Autodesk Fusion 360 part; units mm, degrees
(part 2 of 2)
  arc A367 (268.1669, -101.5666) -> (267.6669, -101.0666) centre (267.6669, -101.5666) ccw
  arc A368 (269.9703, -102.354) -> (269.4703, -101.854) centre (269.4703, -102.354) ccw
  arc A369 (269.9703, -102.5224) -> (270.4703, -103.0224) centre (270.4703, -102.5224) ccw
  arc A370 (272.5183, -103.0224) -> (273.0183, -102.5224) centre (272.5183, -102.5224) ccw
  arc A371 (273.5183, -101.854) -> (273.0183, -102.354) centre (273.5183, -102.354) ccw
  arc A372 (274.3216, -101.854) -> (274.8216, -101.354) centre (274.3216, -101.354) ccw
  arc A373 (275.3216, -95.758) -> (274.8216, -96.258) centre (275.3216, -96.258) ccw
  arc A374 (275.6852, -93.464) -> (275.1852, -92.964) centre (275.1852, -93.464) ccw
  arc A375 (274.8216, -90.0604) -> (274.3216, -89.5604) centre (274.3216, -90.0604) ccw
  line L406 (293.5375, -88.25) -> (306.5375, -88.25)
  line L407 (293.5375, -102.25) -> (306.5375, -102.25)
  line L408 (293.0375, -88.75) -> (293.0375, -101.75)
  line L409 (307.0375, -88.75) -> (307.0375, -101.75)
  arc A376 (293.5375, -88.25) -> (293.0375, -88.75) centre (293.5375, -88.75) ccw
  arc A377 (307.0375, -88.75) -> (306.5375, -88.25) centre (306.5375, -88.75) ccw
  arc A378 (293.0375, -101.75) -> (293.5375, -102.25) centre (293.5375, -101.75) ccw
  arc A379 (306.5375, -102.25) -> (307.0375, -101.75) centre (306.5375, -101.75) ccw
  line L410 (312.5875, -88.25) -> (325.5875, -88.25)
  line L411 (312.5875, -102.25) -> (325.5875, -102.25)
  line L412 (312.0875, -88.75) -> (312.0875, -101.75)
  line L413 (326.0875, -88.75) -> (326.0875, -101.75)
  arc A380 (312.5875, -88.25) -> (312.0875, -88.75) centre (312.5875, -88.75) ccw
  arc A381 (326.0875, -88.75) -> (325.5875, -88.25) centre (325.5875, -88.75) ccw
  arc A382 (312.0875, -101.75) -> (312.5875, -102.25) centre (312.5875, -101.75) ccw
  arc A383 (325.5875, -102.25) -> (326.0875, -101.75) centre (325.5875, -101.75) ccw
  line L414 (331.6375, -88.25) -> (344.6375, -88.25)
  line L415 (331.6375, -102.25) -> (344.6375, -102.25)
  line L416 (331.1375, -88.75) -> (331.1375, -101.75)
  line L417 (345.1375, -88.75) -> (345.1375, -101.75)
  arc A384 (331.6375, -88.25) -> (331.1375, -88.75) centre (331.6375, -88.75) ccw
  arc A385 (345.1375, -88.75) -> (344.6375, -88.25) centre (344.6375, -88.75) ccw
  arc A386 (331.1375, -101.75) -> (331.6375, -102.25) centre (331.6375, -101.75) ccw
  arc A387 (344.6375, -102.25) -> (345.1375, -101.75) centre (344.6375, -101.75) ccw
  line L418 (5.4062, -107.3) -> (18.4063, -107.3)
  line L419 (5.4062, -121.3) -> (18.4063, -121.3)
  line L420 (4.9062, -107.8) -> (4.9062, -120.8)
  line L421 (18.9062, -107.8) -> (18.9062, -120.8)
  arc A388 (5.4062, -107.3) -> (4.9062, -107.8) centre (5.4062, -107.8) ccw
  arc A389 (18.9062, -107.8) -> (18.4062, -107.3) centre (18.4062, -107.8) ccw
  arc A390 (4.9062, -120.8) -> (5.4062, -121.3) centre (5.4062, -120.8) ccw
  arc A391 (18.4062, -121.3) -> (18.9063, -120.8) centre (18.4062, -120.8) ccw
  line L422 (29.2188, -107.3) -> (42.2188, -107.3)
  line L423 (29.2188, -121.3) -> (42.2188, -121.3)
  line L424 (28.7188, -107.8) -> (28.7188, -120.8)
  line L425 (42.7188, -107.8) -> (42.7188, -120.8)
  arc A392 (29.2188, -107.3) -> (28.7187, -107.8) centre (29.2188, -107.8) ccw
  arc A393 (42.7188, -107.8) -> (42.2188, -107.3) centre (42.2188, -107.8) ccw
  arc A394 (28.7188, -120.8) -> (29.2188, -121.3) centre (29.2188, -120.8) ccw
  arc A395 (42.2188, -121.3) -> (42.7188, -120.8) centre (42.2188, -120.8) ccw
  line L426 (53.0313, -107.3) -> (66.0312, -107.3)
  line L427 (53.0313, -121.3) -> (66.0312, -121.3)
  line L428 (52.5313, -107.8) -> (52.5313, -120.8)
  line L429 (66.5312, -107.8) -> (66.5312, -120.8)
  arc A396 (53.0313, -107.3) -> (52.5312, -107.8) centre (53.0313, -107.8) ccw
  arc A397 (66.5312, -107.8) -> (66.0312, -107.3) centre (66.0312, -107.8) ccw
  arc A398 (52.5313, -120.8) -> (53.0313, -121.3) centre (53.0313, -120.8) ccw
  arc A399 (66.0312, -121.3) -> (66.5312, -120.8) centre (66.0312, -120.8) ccw
  line L430 (124.4688, -107.3) -> (137.4688, -107.3)
  line L431 (124.4688, -121.3) -> (137.4688, -121.3)
  line L432 (123.9688, -107.8) -> (123.9688, -120.8)
  line L433 (137.9688, -107.8) -> (137.9688, -120.8)
  arc A400 (124.4688, -107.3) -> (123.9688, -107.8) centre (124.4688, -107.8) ccw
  arc A401 (137.9688, -107.8) -> (137.4688, -107.3) centre (137.4688, -107.8) ccw
  arc A402 (123.9688, -120.8) -> (124.4688, -121.3) centre (124.4688, -120.8) ccw
  arc A403 (137.4688, -121.3) -> (137.9688, -120.8) centre (137.4688, -120.8) ccw
  line L434 (78.1414, -108.6104) -> (83.7961, -108.6104)
  line L435 (84.2961, -109.1104) -> (84.2961, -111.5)
  line L436 (84.7962, -112) -> (130.9688, -112)
  line L437 (130.9688, -116.6) -> (84.7961, -116.6)
  line L438 (84.2961, -117.1) -> (84.2961, -120.404)
  line L439 (83.7961, -120.904) -> (82.9928, -120.904)
  line L440 (82.4928, -121.404) -> (82.4928, -121.5724)
  line L441 (81.9928, -122.0724) -> (79.9447, -122.0724)
  line L442 (79.4447, -121.5724) -> (79.4447, -121.404)
  line L443 (78.9447, -120.904) -> (78.1414, -120.904)
  line L444 (77.6414, -120.404) -> (77.6414, -115.308)
  line L445 (77.1414, -114.808) -> (76.7777, -114.808)
  line L446 (76.7777, -114.808) -> (76.7777, -112.514)
  line L447 (77.2777, -112.014) -> (77.6414, -112.014)
  line L448 (77.6414, -112.014) -> (77.6414, -109.1104)
  arc A404 (84.2962, -109.1104) -> (83.7961, -108.6104) centre (83.7961, -109.1104) ccw
  arc A405 (84.2962, -111.5) -> (84.7962, -112) centre (84.7962, -111.5) ccw
  arc A406 (84.7962, -116.6) -> (84.2962, -117.1) centre (84.7962, -117.1) ccw
  arc A407 (83.7961, -120.904) -> (84.2962, -120.404) centre (83.7961, -120.404) ccw
  arc A408 (82.9928, -120.904) -> (82.4928, -121.404) centre (82.9928, -121.404) ccw
  arc A409 (81.9928, -122.0724) -> (82.4927, -121.5724) centre (81.9928, -121.5724) ccw
  arc A410 (79.4447, -121.5724) -> (79.9447, -122.0724) centre (79.9447, -121.5724) ccw
  arc A411 (79.4447, -121.404) -> (78.9447, -120.904) centre (78.9447, -121.404) ccw
  arc A412 (77.6414, -120.404) -> (78.1414, -120.904) centre (78.1414, -120.404) ccw
  arc A413 (77.6414, -115.308) -> (77.1414, -114.808) centre (77.1414, -115.308) ccw
  arc A414 (77.2777, -112.014) -> (76.7777, -112.514) centre (77.2777, -112.514) ccw
  arc A415 (78.1414, -108.6104) -> (77.6414, -109.1104) centre (78.1414, -109.1104) ccw
  line L449 (183.7962, -108.6104) -> (178.1413, -108.6104)
  line L450 (177.6413, -109.1104) -> (177.6413, -111.5)
  line L451 (177.1413, -112) -> (130.9688, -112)
  line L452 (130.9688, -116.6) -> (177.1413, -116.6)
  line L453 (177.6413, -117.1) -> (177.6413, -120.404)
  line L454 (178.1413, -120.904) -> (178.9447, -120.904)
  line L455 (179.4447, -121.404) -> (179.4447, -121.5724)
  line L456 (179.9447, -122.0724) -> (181.9928, -122.0724)
  line L457 (182.4928, -121.5724) -> (182.4928, -121.404)
  line L458 (182.9928, -120.904) -> (183.7962, -120.904)
  line L459 (184.2962, -120.404) -> (184.2962, -115.308)
  line L460 (184.7962, -114.808) -> (185.1598, -114.808)
  line L461 (185.1598, -114.808) -> (185.1598, -112.514)
  line L462 (184.6598, -112.014) -> (184.2962, -112.014)
  line L463 (184.2962, -112.014) -> (184.2962, -109.1104)
  arc A416 (178.1413, -108.6104) -> (177.6413, -109.1104) centre (178.1413, -109.1104) ccw
  arc A417 (177.1413, -112) -> (177.6413, -111.5) centre (177.1413, -111.5) ccw
  arc A418 (177.6413, -117.1) -> (177.1413, -116.6) centre (177.1413, -117.1) ccw
  arc A419 (177.6413, -120.404) -> (178.1413, -120.904) centre (178.1413, -120.404) ccw
  arc A420 (179.4447, -121.404) -> (178.9447, -120.904) centre (178.9447, -121.404) ccw
  arc A421 (179.4447, -121.5724) -> (179.9447, -122.0724) centre (179.9447, -121.5724) ccw
  arc A422 (181.9928, -122.0724) -> (182.4928, -121.5724) centre (181.9928, -121.5724) ccw
  arc A423 (182.9928, -120.904) -> (182.4928, -121.404) centre (182.9928, -121.404) ccw
  arc A424 (183.7962, -120.904) -> (184.2962, -120.404) centre (183.7962, -120.404) ccw
  arc A425 (184.7962, -114.808) -> (184.2962, -115.308) centre (184.7962, -115.308) ccw
  arc A426 (185.1598, -112.514) -> (184.6598, -112.014) centre (184.6598, -112.514) ccw
  arc A427 (184.2962, -109.1104) -> (183.7962, -108.6104) centre (183.7962, -109.1104) ccw
  line L464 (195.9063, -107.3) -> (208.9062, -107.3)
  line L465 (195.9063, -121.3) -> (208.9062, -121.3)
  line L466 (195.4063, -107.8) -> (195.4063, -120.8)
  line L467 (209.4062, -107.8) -> (209.4062, -120.8)
  arc A428 (195.9063, -107.3) -> (195.4063, -107.8) centre (195.9063, -107.8) ccw
  arc A429 (209.4062, -107.8) -> (208.9062, -107.3) centre (208.9062, -107.8) ccw
  arc A430 (195.4063, -120.8) -> (195.9063, -121.3) centre (195.9063, -120.8) ccw
  arc A431 (208.9062, -121.3) -> (209.4062, -120.8) centre (208.9062, -120.8) ccw
  line L468 (219.7188, -107.3) -> (232.7188, -107.3)
  line L469 (219.7188, -121.3) -> (232.7188, -121.3)
  line L470 (219.2188, -107.8) -> (219.2188, -120.8)
  line L471 (233.2188, -107.8) -> (233.2188, -120.8)
  arc A432 (219.7188, -107.3) -> (219.2188, -107.8) centre (219.7188, -107.8) ccw
  arc A433 (233.2188, -107.8) -> (232.7188, -107.3) centre (232.7188, -107.8) ccw
  arc A434 (219.2188, -120.8) -> (219.7188, -121.3) centre (219.7188, -120.8) ccw
  arc A435 (232.7188, -121.3) -> (233.2188, -120.8) centre (232.7188, -120.8) ccw
  line L472 (243.5313, -107.3) -> (256.5313, -107.3)
  line L473 (243.5313, -121.3) -> (256.5313, -121.3)
  line L474 (243.0312, -107.8) -> (243.0312, -120.8)
  line L475 (257.0312, -107.8) -> (257.0312, -120.8)
  arc A436 (243.5313, -107.3) -> (243.0313, -107.8) centre (243.5313, -107.8) ccw
  arc A437 (257.0312, -107.8) -> (256.5312, -107.3) centre (256.5312, -107.8) ccw
  arc A438 (243.0313, -120.8) -> (243.5313, -121.3) centre (243.5313, -120.8) ccw
  arc A439 (256.5312, -121.3) -> (257.0312, -120.8) centre (256.5312, -120.8) ccw
  line L476 (267.3438, -107.3) -> (280.3438, -107.3)
  line L477 (267.3438, -121.3) -> (280.3438, -121.3)
  line L478 (266.8438, -107.8) -> (266.8438, -120.8)
  line L479 (280.8438, -107.8) -> (280.8438, -120.8)
  arc A440 (267.3438, -107.3) -> (266.8438, -107.8) centre (267.3438, -107.8) ccw
  arc A441 (280.8438, -107.8) -> (280.3438, -107.3) centre (280.3438, -107.8) ccw
  arc A442 (266.8438, -120.8) -> (267.3438, -121.3) centre (267.3438, -120.8) ccw
  arc A443 (280.3438, -121.3) -> (280.8438, -120.8) centre (280.3438, -120.8) ccw
  line L480 (293.5375, -107.3) -> (306.5375, -107.3)
  line L481 (293.5375, -121.3) -> (306.5375, -121.3)
  line L482 (293.0375, -107.8) -> (293.0375, -120.8)
  line L483 (307.0375, -107.8) -> (307.0375, -120.8)
  arc A444 (293.5375, -107.3) -> (293.0375, -107.8) centre (293.5375, -107.8) ccw
  arc A445 (307.0375, -107.8) -> (306.5375, -107.3) centre (306.5375, -107.8) ccw
  arc A446 (293.0375, -120.8) -> (293.5375, -121.3) centre (293.5375, -120.8) ccw
  arc A447 (306.5375, -121.3) -> (307.0375, -120.8) centre (306.5375, -120.8) ccw
  line L484 (312.5875, -107.3) -> (325.5875, -107.3)
  line L485 (312.5875, -121.3) -> (325.5875, -121.3)
  line L486 (312.0875, -107.8) -> (312.0875, -120.8)
  line L487 (326.0875, -107.8) -> (326.0875, -120.8)
  arc A448 (312.5875, -107.3) -> (312.0875, -107.8) centre (312.5875, -107.8) ccw
  arc A449 (326.0875, -107.8) -> (325.5875, -107.3) centre (325.5875, -107.8) ccw
  arc A450 (312.0875, -120.8) -> (312.5875, -121.3) centre (312.5875, -120.8) ccw
  arc A451 (325.5875, -121.3) -> (326.0875, -120.8) centre (325.5875, -120.8) ccw
  line L488 (331.6375, -107.3) -> (344.6375, -107.3)
  line L489 (331.6375, -121.3) -> (344.6375, -121.3)
  line L490 (331.1375, -107.8) -> (331.1375, -120.8)
  line L491 (345.1375, -107.8) -> (345.1375, -120.8)
  arc A452 (331.6375, -107.3) -> (331.1375, -107.8) centre (331.6375, -107.8) ccw
  arc A453 (345.1375, -107.8) -> (344.6375, -107.3) centre (344.6375, -107.8) ccw
  arc A454 (331.1375, -120.8) -> (331.6375, -121.3) centre (331.6375, -120.8) ccw
  arc A455 (344.6375, -121.3) -> (345.1375, -120.8) centre (344.6375, -120.8) ccw
  line L492 (0, -123.825) -> (347.6625, -123.825)
  line L493 (0, 0) -> (347.6625, 0)
  line L494 (0, -123.825) -> (0, 0)
  line L495 (347.6625, -123.825) -> (347.6625, 0)
extrude "Extrude1" add sketch "plate-2026-02-23T17_51_34.543Z" along normal blind 1.5
extrude "Extrude2" add 1 faces at (0, 0.5, 82.55) along direction (-1, 0, 0) blind 2
extrude "Extrude3" add 1 faces at (114.5542, 1, 123.825) along direction (0, 0, 1) blind 4
extrude "Extrude4" add 1 faces at (347.6625, 0.5, 42.6083) along direction (1, 0, 0) blind 31.5
extrude "Extrude5" add 1 faces at (252.1083, 1, 0) along direction (0, 0, -1) blind 3
extrude "Extrude6" add 1 faces at (125.0542, 0.5, 127.825) along direction (0, 0, 1) blind 1
